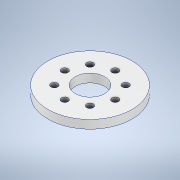
# Autodesk Inventor part: Orifice Plate
Saved by Autodesk Inventor 2021 (Build 250183000, 183)
## iProperties
Created: 2022-07-06
Part Number: Orifice Plate
Material: Aluminum 6061
Document SubType Name: Modeling
Designer: pc
Density: 2.7 g/cm^3
Appearance: Aluminum - Flat
Mass: 175.223 g
Surface Area: 192.313 cm^2
Volume: 64.8975 cm^3
Author: pc
Autodesk Inventor part; units mm, degrees
ref_plane "YZ Plane" through (0, 0, 0) normal (1, 0, 0) x (0, 1, 0)
ref_plane "XZ Plane" through (0, 0, 0) normal (0, 1, 0) x (-1, 0, 0)
ref_plane "XY Plane" through (0, 0, 0) normal (0, 0, 1) x (1, 0, 0)
sketch "Sketch1" plane through (0, 0, 0) normal (0, 1, 0) x (-1, 0, 0)
  circle A0 centre (0, 0) radius 50
  dimension "d1" = 100
  constraints: 1 centre point, 1 coincident
  measures "d1" diameter of A0
extrude "Extrusion1" add sketch "Sketch1" along normal blind 10
sketch "Sketch2" plane through (0, 10, 0) normal (0, 1, 0) x (1, 0, 0)
  circle A0 centre (0, 0) radius 16
  dimension "d4" = 32
  constraints: 1 centre point, 1 coincident
  measures "d4" diameter of A0
hole "Hole1" at (0, 10, 0) direction (0, -1, 0) diameter 35 end through all
sketch "Sketch3" plane through (0, 10, 0) normal (0, 1, 0) x (1, 0, 0)
  circle A0 centre (0, 30) radius 4
  circle A1 centre (-21.2132, 21.2132) radius 4
  circle A2 centre (-30, 0) radius 4
  circle A3 centre (-21.2132, -21.2132) radius 4
  circle A4 centre (0, -30) radius 4
  circle A5 centre (21.2132, -21.2132) radius 4
  circle A6 centre (30, 0) radius 4
  circle A7 centre (21.2132, 21.2132) radius 4
  point P0 (0, 0)
  point P1 (0, 0)
  dimension "d12" = 8
  dimension "d13" = 30
  dimension "d16" = 360
  constraints: 8 centre point, 1 coincident, 17 other
  measures "d12" diameter of A0
  measures "d13" distance of A0.centre point (0, 0)
hole "Hole2" at (-21.2132, 10, 21.2132) at (-30, 10, 0) at (-21.2132, 10, -21.2132) at (0, 10, -30) at (21.2132, 10, -21.2132) at (30, 10, 0) at (21.2132, 10, 21.2132) at (0, 10, 30) direction (0, -1, 0) diameter 8 end through all
sketch "Sketch4" plane through (0, 10, 0) normal (0, 1, 0) x (1, 0, 0)
  point P0 (0, 0)
body "Solid1"
